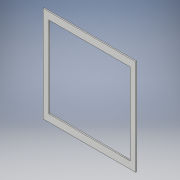
# Autodesk Inventor part: window outer
Saved by Autodesk Inventor 2017 (Build 210142000, 142)
## iProperties
Created: 2019-05-07
Part Number: window outer
Material: Generic
Document SubType Name: Modeling
Designer: Roman
Density: 1 g/cm^3
Appearance: Default
Author: Roman
Autodesk Inventor part; units mm, degrees
ref_plane "YZ Plane" through (0, 0, 0) normal (1, 0, 0) x (0, 1, 0)
ref_plane "XZ Plane" through (0, 0, 0) normal (0, 1, 0) x (-1, 0, 0)
ref_plane "XY Plane" through (0, 0, 0) normal (0, 0, 1) x (1, 0, 0)
sketch "Sketch1" plane through (0, 0, 0) normal (0, 0, 1) x (1, 0, 0)
  line L0 (0, 0) -> (491.0582, 0)
  line L1 (491.0582, 0) -> (491.0582, 508)
  line L2 (491.0582, 508) -> (0, 508)
  line L3 (0, 508) -> (0, 0)
  dimension "d0" = 491.0582
  dimension "d1" = 508
  constraints: 8 end point, 2 parallel, 1 horizontal, 1 perpendicular
  measures "d0" distance of L2.end L1.end
  measures "d1" distance of L1.end L0.end
extrude "Extrusion1" add sketch "Sketch1" along normal blind 6.35
sketch "Sketch2" plane through (0, 0, 6.35) normal (0, 0, 1) x (1, 0, 0)
  line L0 (29.6291, 469.9) -> (461.4291, 469.9)
  line L1 (461.4291, 469.9) -> (461.4291, 38.1)
  line L2 (461.4291, 38.1) -> (29.6291, 38.1)
  line L3 (29.6291, 38.1) -> (29.6291, 469.9)
  line L4 (245.5291, 38.1) -> (245.5291, 0)
  line L5 (0, 0) -> (491.0582, 0) projected
  line L6 (245.5291, 469.9) -> (245.5291, 508)
  line L7 (491.0582, 508) -> (0, 508) projected
  line L8 (29.6291, 254) -> (0, 254)
  line L9 (0, 508) -> (0, 0) projected
  line L10 (461.4291, 254) -> (491.0582, 254)
  line L11 (491.0582, 0) -> (491.0582, 508) projected
  dimension "d4" = 431.8
  dimension "d5" = 431.8
  constraints: 16 end point, 8 midpoint, 2 collinear, 2 parallel, 1 horizontal, 1 perpendicular
  measures "d4" distance between parallel lines of L1 L3
  measures "d5" distance between parallel lines of L0 L2
extrude "Extrusion2" cut sketch "Sketch2" against normal blind 6.35 contours L0 L1 L2 L3
body "Solid1"
